Autodesk Inventor part; units mm, degrees
(part 2 of 4)
  line L562 (14.440387, 25.9675) -> (14.40122, 25.911667)
  line L563 (14.40122, 25.911667) -> (14.362054, 25.855)
  line L564 (14.362054, 25.855) -> (14.288721, 25.781667)
  line L565 (14.288721, 25.781667) -> (14.216221, 25.708334)
  line L566 (14.216221, 25.708334) -> (14.165388, 25.673334)
  line L567 (14.165388, 25.673334) -> (14.113721, 25.639168)
  line L568 (14.113721, 25.639168) -> (14.070388, 25.613335)
  line L569 (14.070388, 25.613335) -> (14.026222, 25.587501)
  line L570 (14.026222, 25.587501) -> (13.940389, 25.550835)
  line L571 (13.940389, 25.550835) -> (13.854556, 25.514168)
  line L572 (13.854556, 25.514168) -> (13.808722, 25.500835)
  line L573 (13.808722, 25.500835) -> (13.762056, 25.487501)
  line L574 (13.762056, 25.487501) -> (13.762056, 25.481668)
  line L575 (13.762056, 25.481668) -> (13.762056, 25.476668)
  line L576 (13.762056, 25.476668) -> (13.967889, 25.007504)
  line L577 (13.967889, 25.007504) -> (14.174555, 24.539171)
  line L578 (14.174555, 24.539171) -> (14.195388, 24.544171)
  line L579 (14.195388, 24.544171) -> (14.216221, 24.548337)
  line L580 (14.216221, 24.548337) -> (14.353721, 24.594171)
  line L581 (14.353721, 24.594171) -> (14.490387, 24.639171)
  line L582 (14.490387, 24.639171) -> (14.612053, 24.70167)
  line L583 (14.612053, 24.70167) -> (14.732886, 24.763337)
  line L584 (14.732886, 24.763337) -> (14.810386, 24.817503)
  line L585 (14.810386, 24.817503) -> (14.887052, 24.87167)
  line L586 (14.887052, 24.87167) -> (15.010385, 24.995003)
  line L587 (15.010385, 24.995003) -> (15.132885, 25.117502)
  line L588 (15.132885, 25.117502) -> (15.187885, 25.195002)
  line L589 (15.187885, 25.195002) -> (15.242051, 25.272502)
  line L590 (15.242051, 25.272502) -> (15.290384, 25.359168)
  line L591 (15.290384, 25.359168) -> (15.338717, 25.445834)
  line L592 (15.338717, 25.445834) -> (15.379551, 25.5475)
  line L593 (15.379551, 25.5475) -> (15.421217, 25.649167)
  line L594 (15.421217, 25.649167) -> (15.44955, 25.749999)
  line L595 (15.44955, 25.749999) -> (15.478717, 25.850832)
  line L596 (15.478717, 25.850832) -> (15.495383, 25.928332)
  line L597 (15.495383, 25.928332) -> (15.51205, 26.004998)
  line L598 (15.51205, 26.004998) -> (15.526217, 26.111665)
  line L599 (15.526217, 26.111665) -> (15.540383, 26.217497)
  line L600 (15.540383, 26.217497) -> (15.541217, 26.484163)
  line L601 (15.541217, 26.484163) -> (15.541217, 26.750829)
  line L602 (15.541217, 26.750829) -> (15.530383, 26.838329)
  line L603 (15.530383, 26.838329) -> (15.520383, 26.925829)
  line L604 (15.520383, 26.925829) -> (15.498717, 27.045828)
  line L605 (15.498717, 27.045828) -> (15.47705, 27.166661)
  line L606 (15.47705, 27.166661) -> (15.448717, 27.264994)
  line L607 (15.448717, 27.264994) -> (15.420384, 27.363327)
  line L608 (15.420384, 27.363327) -> (15.375384, 27.475827)
  line L609 (15.375384, 27.475827) -> (15.330384, 27.58916)
  line L610 (15.330384, 27.58916) -> (15.278717, 27.67916)
  line L611 (15.278717, 27.67916) -> (15.227051, 27.769993)
  line L612 (15.227051, 27.769993) -> (15.173718, 27.841659)
  line L613 (15.173718, 27.841659) -> (15.120385, 27.913325)
  line L614 (15.120385, 27.913325) -> (15.061218, 27.975825)
  line L615 (15.061218, 27.975825) -> (15.001218, 28.038325)
  line L616 (15.001218, 28.038325) -> (14.925385, 28.099158)
  line L617 (14.925385, 28.099158) -> (14.849552, 28.159991)
  line L618 (14.849552, 28.159991) -> (14.795385, 28.194158)
  line L619 (14.795385, 28.194158) -> (14.741219, 28.228324)
  line L620 (14.741219, 28.228324) -> (14.663719, 28.266657)
  line L621 (14.663719, 28.266657) -> (14.587053, 28.304991)
  line L622 (14.587053, 28.304991) -> (14.510387, 28.333324)
  line L623 (14.510387, 28.333324) -> (14.432887, 28.361657)
  line L624 (14.432887, 28.361657) -> (14.343721, 28.383324)
  line L625 (14.343721, 28.383324) -> (14.253721, 28.40499)
  line L626 (14.253721, 28.40499) -> (14.172054, 28.418324)
  line L627 (14.172054, 28.418324) -> (14.091221, 28.43249)
  line L628 (14.091221, 28.43249) -> (13.768721, 28.435823)
  line L629 (13.768721, 28.435823) -> (13.447056, 28.43999)
  line L630 (13.447056, 28.43999) -> (13.347889, 28.430823)
  line L631 (13.347889, 28.430823) -> (13.249556, 28.421657)
  line L632 (13.249556, 28.421657) -> (13.17039, 28.408324)
  line L633 (13.17039, 28.408324) -> (13.091223, 28.39499)
  line L634 (13.091223, 28.39499) -> (12.99539, 28.365824)
  line L635 (12.99539, 28.365824) -> (12.899557, 28.33749)
  line L636 (12.899557, 28.33749) -> (12.832891, 28.307491)
  line L637 (12.832891, 28.307491) -> (12.766225, 28.277491)
  line L638 (12.766225, 28.277491) -> (12.702058, 28.237491)
  line L639 (12.702058, 28.237491) -> (12.637892, 28.197491)
  line L640 (12.637892, 28.197491) -> (12.568725, 28.144991)
  line L641 (12.568725, 28.144991) -> (12.499559, 28.093325)
  line L642 (12.499559, 28.093325) -> (12.422059, 28.013325)
  line L643 (12.422059, 28.013325) -> (12.343726, 27.934158)
  line L644 (12.343726, 27.934158) -> (12.290393, 27.859159)
  line L645 (12.290393, 27.859159) -> (12.23706, 27.784159)
  line L646 (12.23706, 27.784159) -> (12.167893, 27.646659)
  line L647 (12.167893, 27.646659) -> (12.098727, 27.50916)
  line L648 (12.098727, 27.50916) -> (12.038727, 27.35916)
  line L649 (12.038727, 27.35916) -> (11.979561, 27.209161)
  line L650 (11.979561, 27.209161) -> (11.927894, 27.050828)
  line L651 (11.927894, 27.050828) -> (11.876228, 26.892495)
  line L652 (11.876228, 26.892495) -> (11.835395, 26.761662)
  line L653 (11.835395, 26.761662) -> (11.795395, 26.629996)
  line L654 (11.795395, 26.629996) -> (11.747895, 26.486663)
  line L655 (11.747895, 26.486663) -> (11.701229, 26.342497)
  line L656 (11.701229, 26.342497) -> (11.657895, 26.236664)
  line L657 (11.657895, 26.236664) -> (11.614562, 26.131664)
  line L658 (11.614562, 26.131664) -> (11.579562, 26.069998)
  line L659 (11.579562, 26.069998) -> (11.543729, 26.007498)
  line L660 (11.543729, 26.007498) -> (11.501229, 25.954165)
  line L661 (11.501229, 25.954165) -> (11.457896, 25.899998)
  line L662 (11.457896, 25.899998) -> (11.397063, 25.844999)
  line L663 (11.397063, 25.844999) -> (11.337063, 25.789165)
  line L664 (11.337063, 25.789165) -> (11.270397, 25.755832)
  line L665 (11.270397, 25.755832) -> (11.204563, 25.723332)
  line L666 (11.204563, 25.723332) -> (11.139563, 25.707499)
  line L667 (11.139563, 25.707499) -> (11.074564, 25.692499)
  line L668 (11.074564, 25.692499) -> (10.853731, 25.693332)
  line L669 (10.853731, 25.693332) -> (10.632898, 25.694166)
  line L670 (10.632898, 25.694166) -> (10.566232, 25.712499)
  line L671 (10.566232, 25.712499) -> (10.500399, 25.729999)
  line L672 (10.500399, 25.729999) -> (10.441232, 25.759999)
  line L673 (10.441232, 25.759999) -> (10.382899, 25.789999)
  line L674 (10.382899, 25.789999) -> (10.345399, 25.819999)
  line L675 (10.345399, 25.819999) -> (10.3079, 25.849999)
  line L676 (10.3079, 25.849999) -> (10.283733, 25.875832)
  line L677 (10.283733, 25.875832) -> (10.259566, 25.900832)
  line L678 (10.259566, 25.900832) -> (10.228733, 25.943332)
  line L679 (10.228733, 25.943332) -> (10.197067, 25.984998)
  line L680 (10.197067, 25.984998) -> (10.171233, 26.036665)
  line L681 (10.171233, 26.036665) -> (10.144567, 26.089164)
  line L682 (10.144567, 26.089164) -> (10.121233, 26.161664)
  line L683 (10.121233, 26.161664) -> (10.097067, 26.234164)
  line L684 (10.097067, 26.234164) -> (10.082067, 26.317497)
  line L685 (10.082067, 26.317497) -> (10.067067, 26.40083)
  line L686 (10.067067, 26.40083) -> (10.067067, 26.554996)
  line L687 (10.067067, 26.554996) -> (10.067067, 26.709162)
  line L688 (10.067067, 26.709162) -> (10.084567, 26.776662)
  line L689 (10.084567, 26.776662) -> (10.102067, 26.844162)
  line L690 (10.102067, 26.844162) -> (10.1229, 26.894995)
  line L691 (10.1229, 26.894995) -> (10.143733, 26.945828)
  line L692 (10.143733, 26.945828) -> (10.191233, 27.019161)
  line L693 (10.191233, 27.019161) -> (10.238733, 27.092495)
  line L694 (10.238733, 27.092495) -> (10.307066, 27.159161)
  line L695 (10.307066, 27.159161) -> (10.375399, 27.225827)
  line L696 (10.375399, 27.225827) -> (10.439565, 27.269994)
  line L697 (10.439565, 27.269994) -> (10.504565, 27.314994)
  line L698 (10.504565, 27.314994) -> (10.593732, 27.35916)
  line L699 (10.593732, 27.35916) -> (10.682898, 27.403327)
  line L700 (10.682898, 27.403327) -> (10.757898, 27.429993)
  line L701 (10.757898, 27.429993) -> (10.832065, 27.455827)
  line L702 (10.832065, 27.455827) -> (10.835398, 27.45916)
  line L703 (10.835398, 27.45916) -> (10.838731, 27.46166)
  line L704 (10.838731, 27.46166) -> (10.632899, 27.906657)
  line L705 (10.632899, 27.906657) -> (10.427066, 28.350823)
  line L706 (10.427066, 28.350823) -> (10.421233, 28.356657)
  line L707 (10.421233, 28.356657) -> (10.415399, 28.363323)
  line L708 (10.415399, 28.363323) -> (10.342066, 28.34249)
  line L709 (10.342066, 28.34249) -> (10.268733, 28.320823)
  line L710 (10.268733, 28.320823) -> (10.173733, 28.284157)
  line L711 (10.173733, 28.284157) -> (10.078733, 28.246657)
  line L712 (10.078733, 28.246657) -> (9.993734, 28.204157)
  line L713 (9.993734, 28.204157) -> (9.907901, 28.161658)
  line L714 (9.907901, 28.161658) -> (9.837067, 28.114991)
  line L715 (9.837067, 28.114991) -> (9.766234, 28.069158)
  line L716 (9.766234, 28.069158) -> (9.716234, 28.030825)
  line L717 (9.716234, 28.030825) -> (9.666234, 27.992492)
  line L718 (9.666234, 27.992492) -> (9.592068, 27.921658)
  line L719 (9.592068, 27.921658) -> (9.517902, 27.850825)
  line L720 (9.517902, 27.850825) -> (9.474568, 27.795825)
  line L721 (9.474568, 27.795825) -> (9.430402, 27.740825)
  line L722 (9.430402, 27.740825) -> (9.378735, 27.662492)
  line L723 (9.378735, 27.662492) -> (9.327069, 27.584159)
  line L724 (9.327069, 27.584159) -> (9.302903, 27.535826)
  line L725 (9.302903, 27.535826) -> (9.277903, 27.487493)
  line L726 (9.277903, 27.487493) -> (9.241236, 27.397493)
  line L727 (9.241236, 27.397493) -> (9.204569, 27.307493)
  line L728 (9.204569, 27.307493) -> (9.179569, 27.220827)
  line L729 (9.179569, 27.220827) -> (9.154569, 27.134161)
  line L730 (9.154569, 27.134161) -> (9.138736, 27.046661)
  line L731 (9.138736, 27.046661) -> (9.122069, 26.959161)
  line L732 (9.122069, 26.959161) -> (9.112903, 26.871662)
  line L733 (9.112903, 26.871662) -> (9.10457, 26.784162)
  line L734 (9.10457, 26.784162) -> (9.101236, 26.675829)
  line L735 (9.101236, 26.675829) -> (9.101239, 26.675831)
  line L736 (5.926259, 152.354502) -> (5.923571, 152.297378)
  line L737 (5.923571, 152.297378) -> (5.929619, 152.199933)
  line L738 (5.929619, 152.199933) -> (5.934996, 152.102487)
  line L739 (5.934996, 152.102487) -> (5.945076, 152.029906)
  line L740 (5.945076, 152.029906) -> (5.955829, 151.957326)
  line L741 (5.955829, 151.957326) -> (5.97263, 151.880041)
  line L742 (5.97263, 151.880041) -> (5.990103, 151.802757)
  line L743 (5.990103, 151.802757) -> (6.020345, 151.714047)
  line L744 (6.020345, 151.714047) -> (6.050587, 151.625338)
  line L745 (6.050587, 151.625338) -> (6.090237, 151.544693)
  line L746 (6.090237, 151.544693) -> (6.129215, 151.464048)
  line L747 (6.129215, 151.464048) -> (6.182978, 151.383403)
  line L748 (6.182978, 151.383403) -> (6.236742, 151.302758)
  line L749 (6.236742, 151.302758) -> (6.296553, 151.235554)
  line L750 (6.296553, 151.235554) -> (6.357037, 151.168349)
  line L751 (6.357037, 151.168349) -> (6.412144, 151.121307)
  line L752 (6.412144, 151.121307) -> (6.467252, 151.074936)
  line L753 (6.467252, 151.074936) -> (6.518999, 151.037974)
  line L754 (6.518999, 151.037974) -> (6.570746, 151.001683)
  line L755 (6.570746, 151.001683) -> (6.640638, 150.962705)
  line L756 (6.640638, 150.962705) -> (6.711202, 150.923727)
  line L757 (6.711202, 150.923727) -> (6.781767, 150.893485)
  line L758 (6.781767, 150.893485) -> (6.853003, 150.863915)
  line L759 (6.853003, 150.863915) -> (6.906766, 150.847114)
  line L760 (6.906766, 150.847114) -> (6.960529, 150.830313)
  line L761 (6.960529, 150.830313) -> (7.018997, 150.8162)
  line L762 (7.018997, 150.8162) -> (7.078136, 150.802087)
  line L763 (7.078136, 150.802087) -> (7.137276, 150.792007)
  line L764 (7.137276, 150.792007) -> (7.195744, 150.781926)
  line L765 (7.195744, 150.781926) -> (7.266308, 150.773189)
  line L766 (7.266308, 150.773189) -> (7.336872, 150.765125)
  line L767 (7.336872, 150.765125) -> (8.523024, 150.765125)
  line L768 (8.523024, 150.765125) -> (9.709176, 150.765125)
  line L769 (9.709176, 150.765125) -> (9.786461, 150.773862)
  line L770 (9.786461, 150.773862) -> (9.863745, 150.78327)
  line L771 (9.863745, 150.78327) -> (9.93767, 150.796039)
  line L772 (9.93767, 150.796039) -> (10.011594, 150.80948)
  line L773 (10.011594, 150.80948) -> (10.10232, 150.835689)
  line L774 (10.10232, 150.835689) -> (10.193717, 150.861899)
  line L775 (10.193717, 150.861899) -> (10.26697, 150.892813)
  line L776 (10.26697, 150.892813) -> (10.340222, 150.923726)
  line L777 (10.340222, 150.923726) -> (10.389281, 150.949936)
  line L778 (10.389281, 150.949936) -> (10.43834, 150.976817)
  line L779 (10.43834, 150.976817) -> (10.49748, 151.014452)
  line L780 (10.49748, 151.014452) -> (10.555947, 151.052758)
  line L781 (10.555947, 151.052758) -> (10.587533, 151.078296)
  line L782 (10.587533, 151.078296) -> (10.619791, 151.104505)
  line L783 (10.619791, 151.104505) -> (10.661457, 151.141467)
  line L784 (10.661457, 151.141467) -> (10.703796, 151.179102)
  line L785 (10.703796, 151.179102) -> (10.754199, 151.234881)
  line L786 (10.754199, 151.234881) -> (10.804602, 151.29066)
  line L787 (10.804602, 151.29066) -> (10.852989, 151.361225)
  line L788 (10.852989, 151.361225) -> (10.901376, 151.431789)
  line L789 (10.901376, 151.431789) -> (10.93901, 151.503697)
  line L790 (10.93901, 151.503697) -> (10.975972, 151.574934)
  line L791 (10.975972, 151.574934) -> (10.999494, 151.629369)
  line L792 (10.999494, 151.629369) -> (11.022343, 151.684476)
  line L793 (11.022343, 151.684476) -> (11.049897, 151.773857)
  line L794 (11.049897, 151.773857) -> (11.076778, 151.863911)
  line L795 (11.076778, 151.863911) -> (11.090219, 151.934475)
  line L796 (11.090219, 151.934475) -> (11.10366, 152.005039)
  line L797 (11.10366, 152.005039) -> (11.111725, 152.066867)
  line L798 (11.111725, 152.066867) -> (11.120461, 152.129367)
  line L799 (11.120461, 152.129367) -> (11.120461, 152.327619)
  line L800 (11.120461, 152.327619) -> (11.120461, 152.525871)
  line L801 (11.120461, 152.525871) -> (11.105004, 152.620629)
  line L802 (11.105004, 152.620629) -> (11.090219, 152.715386)
  line L803 (11.090219, 152.715386) -> (11.073418, 152.783935)
  line L804 (11.073418, 152.783935) -> (11.056617, 152.851811)
  line L805 (11.056617, 152.851811) -> (11.027047, 152.935816)
  line L806 (11.027047, 152.935816) -> (10.997477, 153.020493)
  line L807 (10.997477, 153.020493) -> (10.957155, 153.102482)
  line L808 (10.957155, 153.102482) -> (10.91616, 153.184471)
  line L809 (10.91616, 153.184471) -> (10.875166, 153.247643)
  line L810 (10.875166, 153.247643) -> (10.833499, 153.311487)
  line L811 (10.833499, 153.311487) -> (10.794521, 153.359202)
  line L812 (10.794521, 153.359202) -> (10.755543, 153.406917)
  line L813 (10.755543, 153.406917) -> (10.706484, 153.455976)
  line L814 (10.706484, 153.455976) -> (10.657425, 153.505035)
  line L815 (10.657425, 153.505035) -> (10.608365, 153.544685)
  line L816 (10.608365, 153.544685) -> (10.559306, 153.584336)
  line L817 (10.559306, 153.584336) -> (10.492774, 153.628018)
  line L818 (10.492774, 153.628018) -> (10.426242, 153.671701)
  line L819 (10.426242, 153.671701) -> (10.334845, 153.715384)
  line L820 (10.334845, 153.715384) -> (10.243447, 153.759066)
  line L821 (10.243447, 153.759066) -> (10.185652, 153.779228)
  line L822 (10.185652, 153.779228) -> (10.127184, 153.799389)
  line L823 (10.127184, 153.799389) -> (10.049228, 153.81955)
  line L824 (10.049228, 153.81955) -> (9.971271, 153.839711)
  line L825 (9.971271, 153.839711) -> (9.908771, 153.849792)
  line L826 (9.908771, 153.849792) -> (9.846944, 153.859872)
  line L827 (9.846944, 153.859872) -> (9.785116, 153.867937)
  line L828 (9.785116, 153.867937) -> (9.722616, 153.876001)
  line L829 (9.722616, 153.876001) -> (8.610388, 153.87869)
  line L830 (8.610388, 153.87869) -> (7.49816, 153.880706)
  line L831 (7.49816, 153.880706) -> (7.373833, 153.873313)
  line L832 (7.373833, 153.873313) -> (7.249505, 153.865921)
  line L833 (7.249505, 153.865921) -> (7.183645, 153.856512)
  line L834 (7.183645, 153.856512) -> (7.117785, 153.846432)
  line L835 (7.117785, 153.846432) -> (7.052597, 153.832319)
  line L836 (7.052597, 153.832319) -> (6.987409, 153.818206)
  line L837 (6.987409, 153.818206) -> (6.913485, 153.794685)
  line L838 (6.913485, 153.794685) -> (6.83956, 153.771163)
  line L839 (6.83956, 153.771163) -> (6.775716, 153.744282)
  line L840 (6.775716, 153.744282) -> (6.711872, 153.718072)
  line L841 (6.711872, 153.718072) -> (6.661469, 153.690518)
  line L842 (6.661469, 153.690518) -> (6.611066, 153.662965)
  line L843 (6.611066, 153.662965) -> (6.553943, 153.626002)
  line L844 (6.553943, 153.626002) -> (6.496819, 153.58904)
  line L845 (6.496819, 153.58904) -> (6.446416, 153.548046)
  line L846 (6.446416, 153.548046) -> (6.396013, 153.507051)
  line L847 (6.396013, 153.507051) -> (6.34561, 153.456648)
  line L848 (6.34561, 153.456648) -> (6.295207, 153.406245)
  line L849 (6.295207, 153.406245) -> (6.254213, 153.355842)
  line L850 (6.254213, 153.355842) -> (6.21389, 153.305439)
  line L851 (6.21389, 153.305439) -> (6.186336, 153.265116)
  line L852 (6.186336, 153.265116) -> (6.159455, 153.224794)
  line L853 (6.159455, 153.224794) -> (6.131229, 153.175735)
  line L854 (6.131229, 153.175735) -> (6.103003, 153.126676)
  line L855 (6.103003, 153.126676) -> (6.069401, 153.052751)
  line L856 (6.069401, 153.052751) -> (6.036471, 152.978155)
  line L857 (6.036471, 152.978155) -> (6.010262, 152.895494)
  line L858 (6.010262, 152.895494) -> (5.984052, 152.813505)
  line L859 (5.984052, 152.813505) -> (5.969267, 152.746973)
  line L860 (5.969267, 152.746973) -> (5.955154, 152.680441)
  line L861 (5.955154, 152.680441) -> (5.945746, 152.613237)
  line L862 (5.945746, 152.613237) -> (5.936337, 152.546033)
  line L863 (5.936337, 152.546033) -> (5.932305, 152.478829)
  line L864 (5.932305, 152.478829) -> (5.928945, 152.411625)
  line L865 (5.928945, 152.411625) -> (5.926257, 152.354501)
  line L866 (5.926257, 152.354501) -> (5.926259, 152.354502)
  line L867 (6.729349, 152.314852) -> (6.728677, 152.41297)
  line L868 (6.728677, 152.41297) -> (6.738757, 152.472781)
  line L869 (6.738757, 152.472781) -> (6.74951, 152.532593)
  line L870 (6.74951, 152.532593) -> (6.766983, 152.586356)
  line L871 (6.766983, 152.586356) -> (6.784456, 152.640119)
  line L872 (6.784456, 152.640119) -> (6.809994, 152.690522)
  line L873 (6.809994, 152.690522) -> (6.836203, 152.740925)
  line L874 (6.836203, 152.740925) -> (6.871821, 152.787968)
  line L875 (6.871821, 152.787968) -> (6.90744, 152.835011)
  line L876 (6.90744, 152.835011) -> (6.955827, 152.876005)
  line L877 (6.955827, 152.876005) -> (7.004886, 152.916328)
  line L878 (7.004886, 152.916328) -> (7.041176, 152.938505)
  line L879 (7.041176, 152.938505) -> (7.077466, 152.960683)
  line L880 (7.077466, 152.960683) -> (7.131229, 152.983532)
  line L881 (7.131229, 152.983532) -> (7.184992, 153.007053)
  line L882 (7.184992, 153.007053) -> (7.248164, 153.023182)
  line L883 (7.248164, 153.023182) -> (7.312008, 153.039311)
  line L884 (7.312008, 153.039311) -> (7.394669, 153.046704)
  line L885 (7.394669, 153.046704) -> (7.478002, 153.054096)
  line L886 (7.478002, 153.054096) -> (8.580149, 153.05208)
  line L887 (8.580149, 153.05208) -> (9.682296, 153.049392)
  line L888 (9.682296, 153.049392) -> (9.739419, 153.037295)
  line L889 (9.739419, 153.037295) -> (9.796543, 153.025871)
  line L890 (9.796543, 153.025871) -> (9.857026, 153.005709)
  line L891 (9.857026, 153.005709) -> (9.91751, 152.985548)
  line L892 (9.91751, 152.985548) -> (9.972618, 152.955978)
  line L893 (9.972618, 152.955978) -> (10.028397, 152.926408)
  line L894 (10.028397, 152.926408) -> (10.067375, 152.896838)
  line L895 (10.067375, 152.896838) -> (10.106354, 152.866597)
  line L896 (10.106354, 152.866597) -> (10.143316, 152.826946)
  line L897 (10.143316, 152.826946) -> (10.180278, 152.786624)
  line L898 (10.180278, 152.786624) -> (10.205144, 152.74899)
  line L899 (10.205144, 152.74899) -> (10.230682, 152.710683)
  line L900 (10.230682, 152.710683) -> (10.253531, 152.662296)
  line L901 (10.253531, 152.662296) -> (10.27638, 152.613237)
  line L902 (10.27638, 152.613237) -> (10.293181, 152.555442)
  line L903 (10.293181, 152.555442) -> (10.309982, 152.497646)
  line L904 (10.309982, 152.497646) -> (10.318047, 152.427754)
  line L905 (10.318047, 152.427754) -> (10.326111, 152.357862)
  line L906 (10.326111, 152.357862) -> (10.321407, 152.272513)
  line L907 (10.321407, 152.272513) -> (10.317375, 152.186492)
  line L908 (10.317375, 152.186492) -> (10.307294, 152.138105)
  line L909 (10.307294, 152.138105) -> (10.296542, 152.089046)
  line L910 (10.296542, 152.089046) -> (10.283773, 152.052083)
  line L911 (10.283773, 152.052083) -> (10.271004, 152.015121)
  line L912 (10.271004, 152.015121) -> (10.250843, 151.972783)
  line L913 (10.250843, 151.972783) -> (10.230009, 151.931116)
  line L914 (10.230009, 151.931116) -> (10.199096, 151.884073)
  line L915 (10.199096, 151.884073) -> (10.168182, 151.83703)
  line L916 (10.168182, 151.83703) -> (10.117779, 151.789316)
  line L917 (10.117779, 151.789316) -> (10.068048, 151.742273)
  line L918 (10.068048, 151.742273) -> (10.019661, 151.711359)
  line L919 (10.019661, 151.711359) -> (9.971946, 151.679773)
  line L920 (9.971946, 151.679773) -> (9.918183, 151.657596)
  line L921 (9.918183, 151.657596) -> (9.863748, 151.634746)
  line L922 (9.863748, 151.634746) -> (9.826785, 151.624666)
  line L923 (9.826785, 151.624666) -> (9.790495, 151.613913)
  line L924 (9.790495, 151.613913) -> (9.73942, 151.60316)
  line L925 (9.73942, 151.60316) -> (9.689017, 151.592408)
  line L926 (9.689017, 151.592408) -> (8.573429, 151.590392)
  line L927 (8.573429, 151.590392) -> (7.45784, 151.587703)
  line L928 (7.45784, 151.587703) -> (7.385932, 151.595096)
  line L929 (7.385932, 151.595096) -> (7.314023, 151.602488)
  line L930 (7.314023, 151.602488) -> (7.244803, 151.619289)
  line L931 (7.244803, 151.619289) -> (7.175583, 151.636762)
  line L932 (7.175583, 151.636762) -> (7.114427, 151.66566)
  line L933 (7.114427, 151.66566) -> (7.053272, 151.694558)
  line L934 (7.053272, 151.694558) -> (7.013621, 151.720768)
  line L935 (7.013621, 151.720768) -> (6.973971, 151.747649)
  line L936 (6.973971, 151.747649) -> (6.938353, 151.779907)
  line L937 (6.938353, 151.779907) -> (6.902734, 151.812165)
  line L938 (6.902734, 151.812165) -> (6.871149, 151.85316)
  line L939 (6.871149, 151.85316) -> (6.839563, 151.894154)
  line L940 (6.839563, 151.894154) -> (6.807977, 151.95531)
  line L941 (6.807977, 151.95531) -> (6.777063, 152.017138)
  line L942 (6.777063, 152.017138) -> (6.76295, 152.062836)
  line L943 (6.76295, 152.062836) -> (6.749509, 152.109207)
  line L944 (6.749509, 152.109207) -> (6.739429, 152.16297)
  line L945 (6.739429, 152.16297) -> (6.73002, 152.216733)
  line L946 (6.73002, 152.216733) -> (6.729348, 152.314851)
  line L947 (6.729348, 152.314851) -> (6.729349, 152.314852)
  line L948 (5.926259, 162.82489) -> (5.924243, 162.761046)
  line L949 (5.924243, 162.761046) -> (5.928947, 162.66696)
  line L950 (5.928947, 162.66696) -> (5.934324, 162.572875)
  line L951 (5.934324, 162.572875) -> (5.945076, 162.497606)
  line L952 (5.945076, 162.497606) -> (5.955829, 162.421666)
  line L953 (5.955829, 162.421666) -> (5.969942, 162.356477)
  line L954 (5.969942, 162.356477) -> (5.984055, 162.290618)
  line L955 (5.984055, 162.290618) -> (6.012952, 162.20258)
  line L956 (6.012952, 162.20258) -> (6.04185, 162.114543)
  line L957 (6.04185, 162.114543) -> (6.077468, 162.038602)
  line L958 (6.077468, 162.038602) -> (6.112415, 161.961989)
  line L959 (6.112415, 161.961989) -> (6.146016, 161.905538)
  line L960 (6.146016, 161.905538) -> (6.179619, 161.848414)
  line L961 (6.179619, 161.848414) -> (6.228678, 161.783226)
  line L962 (6.228678, 161.783226) -> (6.277065, 161.71871)
  line L963 (6.277065, 161.71871) -> (6.343597, 161.65285)
  line L964 (6.343597, 161.65285) -> (6.409457, 161.586318)
  line L965 (6.409457, 161.586318) -> (6.46322, 161.54398)
  line L966 (6.46322, 161.54398) -> (6.517655, 161.502313)
  line L967 (6.517655, 161.502313) -> (6.574107, 161.466695)
  line L968 (6.574107, 161.466695) -> (6.63123, 161.431749)
  line L969 (6.63123, 161.431749) -> (6.701794, 161.396803)
  line L970 (6.701794, 161.396803) -> (6.772359, 161.361857)
  line L971 (6.772359, 161.361857) -> (6.836203, 161.337663)
  line L972 (6.836203, 161.337663) -> (6.900719, 161.31347)
  line L973 (6.900719, 161.31347) -> (6.973971, 161.293309)
  line L974 (6.973971, 161.293309) -> (7.047895, 161.273148)
  line L975 (7.047895, 161.273148) -> (7.1319, 161.259035)
  line L976 (7.1319, 161.259035) -> (7.215906, 161.244922)
  line L977 (7.215906, 161.244922) -> (7.27975, 161.237529)
  line L978 (7.27975, 161.237529) -> (7.343593, 161.230137)
  line L979 (7.343593, 161.230137) -> (8.42222, 161.227449)
  line L980 (8.42222, 161.227449) -> (9.500846, 161.224761)
  line L981 (9.500846, 161.224761) -> (9.645335, 161.232153)
  line L982 (9.645335, 161.232153) -> (9.789823, 161.238873)
  line L983 (9.789823, 161.238873) -> (9.859043, 161.248954)
  line L984 (9.859043, 161.248954) -> (9.928263, 161.259035)
  line L985 (9.928263, 161.259035) -> (10.005548, 161.275836)
  line L986 (10.005548, 161.275836) -> (10.082161, 161.292637)
  line L987 (10.082161, 161.292637) -> (10.16415, 161.319518)
  line L988 (10.16415, 161.319518) -> (10.246811, 161.347072)
  line L989 (10.246811, 161.347072) -> (10.342913, 161.393443)
  line L990 (10.342913, 161.393443) -> (10.438342, 161.440486)
  line L991 (10.438342, 161.440486) -> (10.50017, 161.48148)
  line L992 (10.50017, 161.48148) -> (10.561326, 161.521803)
  line L993 (10.561326, 161.521803) -> (10.611729, 161.563469)
  line L994 (10.611729, 161.563469) -> (10.662132, 161.605135)
  line L995 (10.662132, 161.605135) -> (10.725304, 161.670324)
  line L996 (10.725304, 161.670324) -> (10.787803, 161.736183)
  line L997 (10.787803, 161.736183) -> (10.830814, 161.793979)
  line L998 (10.830814, 161.793979) -> (10.873153, 161.851774)
  line L999 (10.873153, 161.851774) -> (10.914819, 161.923683)
  line L1000 (10.914819, 161.923683) -> (10.955814, 161.995591)
  line L1001 (10.955814, 161.995591) -> (10.986055, 162.064139)
  line L1002 (10.986055, 162.064139) -> (11.016297, 162.132688)
  line L1003 (11.016297, 162.132688) -> (11.03713, 162.198548)
  line L1004 (11.03713, 162.198548) -> (11.057964, 162.263736)
  line L1005 (11.057964, 162.263736) -> (11.074093, 162.326235)
  line L1006 (11.074093, 162.326235) -> (11.090221, 162.388735)
  line L1007 (11.090221, 162.388735) -> (11.105006, 162.484165)
  line L1008 (11.105006, 162.484165) -> (11.120463, 162.579595)
  line L1009 (11.120463, 162.579595) -> (11.120463, 162.771127)
  line L1010 (11.120463, 162.771127) -> (11.120463, 162.962658)
  line L1011 (11.120463, 162.962658) -> (11.109039, 163.053384)
  line L1012 (11.109039, 163.053384) -> (11.096942, 163.144109)
  line L1013 (11.096942, 163.144109) -> (11.078797, 163.221394)
  line L1014 (11.078797, 163.221394) -> (11.05998, 163.298678)
  line L1015 (11.05998, 163.298678) -> (11.035114, 163.376635)
  line L1016 (11.035114, 163.376635) -> (11.010921, 163.455264)
  line L1017 (11.010921, 163.455264) -> (10.97463, 163.531205)
  line L1018 (10.97463, 163.531205) -> (10.93834, 163.607817)
  line L1019 (10.93834, 163.607817) -> (10.910114, 163.656876)
  line L1020 (10.910114, 163.656876) -> (10.881889, 163.705263)
  line L1021 (10.881889, 163.705263) -> (10.846271, 163.754994)
  line L1022 (10.846271, 163.754994) -> (10.811324, 163.804725)
  line L1023 (10.811324, 163.804725) -> (10.769658, 163.854456)
  line L1024 (10.769658, 163.854456) -> (10.728663, 163.903515)
  line L1025 (10.728663, 163.903515) -> (10.658771, 163.966687)
  line L1026 (10.658771, 163.966687) -> (10.589551, 164.029187)
  line L1027 (10.589551, 164.029187) -> (10.510922, 164.082278)
  line L1028 (10.510922, 164.082278) -> (10.431622, 164.135369)
  line L1029 (10.431622, 164.135369) -> (10.349633, 164.17502)
  line L1030 (10.349633, 164.17502) -> (10.266972, 164.215342)
  line L1031 (10.266972, 164.215342) -> (10.201112, 164.239536)
  line L1032 (10.201112, 164.239536) -> (10.135924, 164.263057)
  line L1033 (10.135924, 164.263057) -> (10.058639, 164.283218)
  line L1034 (10.058639, 164.283218) -> (9.981355, 164.30338)
  line L1035 (9.981355, 164.30338) -> (9.90071, 164.31682)
  line L1036 (9.90071, 164.31682) -> (9.820065, 164.330261)
  line L1037 (9.820065, 164.330261) -> (9.724635, 164.337654)
  line L1038 (9.724635, 164.337654) -> (9.628533, 164.344374)
  line L1039 (9.628533, 164.344374) -> (8.459183, 164.341686)
  line L1040 (8.459183, 164.341686) -> (7.289833, 164.338998)
  line L1041 (7.289833, 164.338998) -> (7.217252, 164.327573)
  line L1042 (7.217252, 164.327573) -> (7.144672, 164.31682)
  line L1043 (7.144672, 164.31682) -> (7.064027, 164.300019)
  line L1044 (7.064027, 164.300019) -> (6.984054, 164.283218)
  line L1045 (6.984054, 164.283218) -> (6.888624, 164.251633)
  line L1046 (6.888624, 164.251633) -> (6.793866, 164.220719)
  line L1047 (6.793866, 164.220719) -> (6.701125, 164.174348)
  line L1048 (6.701125, 164.174348) -> (6.607711, 164.128649)
  line L1049 (6.607711, 164.128649) -> (6.542523, 164.084295)
  line L1050 (6.542523, 164.084295) -> (6.476663, 164.03994)
  line L1051 (6.476663, 164.03994) -> (6.4229, 163.994241)
  line L1052 (6.4229, 163.994241) -> (6.369137, 163.948542)
  line L1053 (6.369137, 163.948542) -> (6.328814, 163.905532)
  line L1054 (6.328814, 163.905532) -> (6.28782, 163.863193)
  line L1055 (6.28782, 163.863193) -> (6.250186, 163.816151)
  line L1056 (6.250186, 163.816151) -> (6.213223, 163.769108)
  line L1057 (6.213223, 163.769108) -> (6.179621, 163.718705)
  line L1058 (6.179621, 163.718705) -> (6.145347, 163.668302)
  line L1059 (6.145347, 163.668302) -> (6.115106, 163.611178)
  line L1060 (6.115106, 163.611178) -> (6.084192, 163.554055)
  line L1061 (6.084192, 163.554055) -> (6.053278, 163.48013)
  line L1062 (6.053278, 163.48013) -> (6.022364, 163.406878)
  line L1063 (6.022364, 163.406878) -> (6.000187, 163.329593)
  line L1064 (6.000187, 163.329593) -> (5.977337, 163.251637)
  line L1065 (5.977337, 163.251637) -> (5.963896, 163.181072)
  line L1066 (5.963896, 163.181072) -> (5.949784, 163.110508)
  line L1067 (5.949784, 163.110508) -> (5.943063, 163.063465)
  line L1068 (5.943063, 163.063465) -> (5.936343, 163.016422)
  line L1069 (5.936343, 163.016422) -> (5.932983, 162.952579)
  line L1070 (5.932983, 162.952579) -> (5.92895, 162.888735)
  line L1071 (5.92895, 162.888735) -> (5.926262, 162.824891)
  line L1072 (5.926262, 162.824891) -> (5.926259, 162.82489)
  line L1073 (6.729349, 162.778519) -> (6.728677, 162.876637)
  line L1074 (6.728677, 162.876637) -> (6.738757, 162.936449)
  line L1075 (6.738757, 162.936449) -> (6.74951, 162.996261)
  line L1076 (6.74951, 162.996261) -> (6.763623, 163.043303)
  line L1077 (6.763623, 163.043303) -> (6.777064, 163.090346)
  line L1078 (6.777064, 163.090346) -> (6.805961, 163.14747)
  line L1079 (6.805961, 163.14747) -> (6.834859, 163.204593)
  line L1080 (6.834859, 163.204593) -> (6.866445, 163.24626)
  line L1081 (6.866445, 163.24626) -> (6.898031, 163.288598)
  line L1082 (6.898031, 163.288598) -> (6.944402, 163.330937)
  line L1083 (6.944402, 163.330937) -> (6.990773, 163.373275)
  line L1084 (6.990773, 163.373275) -> (7.043192, 163.404189)
  line L1085 (7.043192, 163.404189) -> (7.094939, 163.435103)
  line L1086 (7.094939, 163.435103) -> (7.155423, 163.458624)
  line L1087 (7.155423, 163.458624) -> (7.215907, 163.482818)
  line L1088 (7.215907, 163.482818) -> (7.283111, 163.498275)
  line L1089 (7.283111, 163.498275) -> (7.350315, 163.51306)
  line L1090 (7.350315, 163.51306) -> (8.479342, 163.515748)
  line L1091 (8.479342, 163.515748) -> (9.60837, 163.517764)
  line L1092 (9.60837, 163.517764) -> (9.674902, 163.510372)
  line L1093 (9.674902, 163.510372) -> (9.742106, 163.502307)
  line L1094 (9.742106, 163.502307) -> (9.803262, 163.48685)
  line L1095 (9.803262, 163.48685) -> (9.864417, 163.471393)
  line L1096 (9.864417, 163.471393) -> (9.916837, 163.449888)
  line L1097 (9.916837, 163.449888) -> (9.968584, 163.428383)
  line L1098 (9.968584, 163.428383) -> (10.020331, 163.394781)
  line L1099 (10.020331, 163.394781) -> (10.072078, 163.360507)
  line L1100 (10.072078, 163.360507) -> (10.117777, 163.316152)
  line L1101 (10.117777, 163.316152) -> (10.164148, 163.271797)
  line L1102 (10.164148, 163.271797) -> (10.193717, 163.230803)
  line L1103 (10.193717, 163.230803) -> (10.223287, 163.189136)
  line L1104 (10.223287, 163.189136) -> (10.253529, 163.12462)
  line L1105 (10.253529, 163.12462) -> (10.283771, 163.060104)
  line L1106 (10.283771, 163.060104) -> (10.297212, 163.006341)
  line L1107 (10.297212, 163.006341) -> (10.310652, 162.952578)
  line L1108 (10.310652, 162.952578) -> (10.317373, 162.89747)
  line L1109 (10.317373, 162.89747) -> (10.324093, 162.842363)
  line L1110 (10.324093, 162.842363) -> (10.324093, 162.784568)
  line L1111 (10.324093, 162.784568) -> (10.324093, 162.726772)
  line L1112 (10.324093, 162.726772) -> (10.317373, 162.672337)
  line L1113 (10.317373, 162.672337) -> (10.310652, 162.617902)
  line L1114 (10.310652, 162.617902) -> (10.297212, 162.566827)
  line L1115 (10.297212, 162.566827) -> (10.284443, 162.516424)
  line L1116 (10.284443, 162.516424) -> (10.26361, 162.465349)
  line L1117 (10.26361, 162.465349) -> (10.242104, 162.414274)
  line L1118 (10.242104, 162.414274) -> (10.210518, 162.365887)
  line L1119 (10.210518, 162.365887) -> (10.17826, 162.3175)
  line L1120 (10.17826, 162.3175) -> (10.14533, 162.281209)
  line L1121 (10.14533, 162.281209) -> (10.1124, 162.244247)
  line L1122 (10.1124, 162.244247) -> (10.058637, 162.204597)
  line L1123 (10.058637, 162.204597) -> (10.004874, 162.164274)
  line L1124 (10.004874, 162.164274) -> (9.942374, 162.134704)
  line L1125 (9.942374, 162.134704) -> (9.880546, 162.105134)
  line L1126 (9.880546, 162.105134) -> (9.803934, 162.085645)
  line L1127 (9.803934, 162.085645) -> (9.727321, 162.066156)
  line L1128 (9.727321, 162.066156) -> (9.647348, 162.059435)
  line L1129 (9.647348, 162.059435) -> (9.568047, 162.052043)
  line L1130 (9.568047, 162.052043) -> (8.523023, 162.052043)
  line L1131 (8.523023, 162.052043) -> (7.477998, 162.052043)
  line L1132 (7.477998, 162.052043) -> (7.400713, 162.058763)
  line L1133 (7.400713, 162.058763) -> (7.323429, 162.065484)
  line L1134 (7.323429, 162.065484) -> (7.255553, 162.082285)
  line L1135 (7.255553, 162.082285) -> (7.187677, 162.099086)
  line L1136 (7.187677, 162.099086) -> (7.14601, 162.115887)
  line L1137 (7.14601, 162.115887) -> (7.104344, 162.132016)
  line L1138 (7.104344, 162.132016) -> (7.060661, 162.156209)
  line L1139 (7.060661, 162.156209) -> (7.01765, 162.180403)
  line L1140 (7.01765, 162.180403) -> (6.96792, 162.220053)
  line L1141 (6.96792, 162.220053) -> (6.91886, 162.259704)
  line L1142 (6.91886, 162.259704) -> (6.885258, 162.30137)
  line L1143 (6.885258, 162.30137) -> (6.851656, 162.342365)
  line L1144 (6.851656, 162.342365) -> (6.822759, 162.392768)
  line L1145 (6.822759, 162.392768) -> (6.793861, 162.443171)
  line L1146 (6.793861, 162.443171) -> (6.771683, 162.507687)
  line L1147 (6.771683, 162.507687) -> (6.749506, 162.572875)
  line L1148 (6.749506, 162.572875) -> (6.739425, 162.626638)
  line L1149 (6.739425, 162.626638) -> (6.730017, 162.680401)
  line L1150 (6.730017, 162.680401) -> (6.729345, 162.778519)
  line L1151 (6.729345, 162.778519) -> (6.729349, 162.778519)
  line L1152 (8.831224, -33.4262) -> (8.829557, -33.806199)
  line L1153 (8.829557, -33.806199) -> (8.868724, -33.819532)
  line L1154 (8.868724, -33.819532) -> (8.908724, -33.832866)
  line L1155 (8.908724, -33.832866) -> (12.008714, -34.778697)
  line L1156 (12.008714, -34.778697) -> (15.108705, -35.725359)
  line L1157 (15.108705, -35.725359) -> (15.132038, -35.730359)
  line L1158 (15.132038, -35.730359) -> (15.154538, -35.735359)
  line L1159 (15.154538, -35.735359) -> (15.152872, -35.207027)
  line L1160 (15.152872, -35.207027) -> (15.150372, -34.678694)
  line L1161 (15.150372, -34.678694) -> (14.575374, -34.522861)
  line L1162 (14.575374, -34.522861) -> (14.000377, -34.367028)
  line L1163 (14.000377, -34.367028) -> (13.98121, -34.362028)
  line L1164 (13.98121, -34.362028) -> (13.962877, -34.357862)
  line L1165 (13.962877, -34.357862) -> (13.962877, -33.426197)
  line L1166 (13.962877, -33.426197) -> (13.962877, -32.494533)
  line L1167 (13.962877, -32.494533) -> (14.544542, -32.337034)
  line L1168 (14.544542, -32.337034) -> (15.125372, -32.180367)
  line L1169 (15.125372, -32.180367) -> (15.139539, -32.172867)
  line L1170 (15.139539, -32.172867) -> (15.154539, -32.165367)
  line L1171 (15.154539, -32.165367) -> (15.154539, -31.645369)
  line L1172 (15.154539, -31.645369) -> (15.154539, -31.12537)
  line L1173 (15.154539, -31.12537) -> (15.148706, -31.122036)
  line L1174 (15.148706, -31.122036) -> (15.142039, -31.118703)
  line L1175 (15.142039, -31.118703) -> (11.987872, -32.082868)
  line L1176 (11.987872, -32.082868) -> (8.833705, -33.046198)
  line L1177 (8.833705, -33.046198) -> (8.831205, -33.426198)
  line L1178 (8.831205, -33.426198) -> (8.831224, -33.4262)
  line L1179 (10.539551, -33.425366) -> (10.550385, -33.4212)
  line L1180 (10.550385, -33.4212) -> (11.779547, -33.087034)
  line L1181 (11.779547, -33.087034) -> (13.00871, -32.752867)
  line L1182 (13.00871, -32.752867) -> (13.01121, -33.423697)
  line L1183 (13.01121, -33.423697) -> (13.012877, -34.093696)
  line L1184 (13.012877, -34.093696) -> (13.010377, -34.096196)
  line L1185 (13.010377, -34.096196) -> (13.007877, -34.099529)
  line L1186 (13.007877, -34.099529) -> (11.76788, -33.764532)
  line L1187 (11.76788, -33.764532) -> (10.527882, -33.429534)
  line L1188 (10.527882, -33.429534) -> (10.539549, -33.425367)
  line L1189 (10.539549, -33.425367) -> (10.539551, -33.425366)
  line L1190 (8.831224, -29.289547) -> (8.829557, -30.44121)
  line L1191 (8.829557, -30.44121) -> (11.987882, -30.44121)
  line L1192 (11.987882, -30.44121) -> (15.146206, -30.44121)
  line L1193 (15.146206, -30.44121) -> (15.146206, -29.941211)
  line L1194 (15.146206, -29.941211) -> (15.146206, -29.441212)
  line L1195 (15.146206, -29.441212) -> (13.829544, -29.441212)
  line L1196 (13.829544, -29.441212) -> (12.512882, -29.441212)
  line L1197 (12.512882, -29.441212) -> (12.512882, -29.05538)
  line L1198 (12.512882, -29.05538) -> (12.512882, -28.670383)
  line L1199 (12.512882, -28.670383) -> (13.829544, -28.124551)
  line L1200 (13.829544, -28.124551) -> (15.145375, -27.578719)
  line L1201 (15.145375, -27.578719) -> (15.146208, -27.004553)
  line L1202 (15.146208, -27.004553) -> (15.146208, -26.431222)
  line L1203 (15.146208, -26.431222) -> (15.133708, -26.436222)
  line L1204 (15.133708, -26.436222) -> (15.121208, -26.441222)
  line L1205 (15.121208, -26.441222) -> (13.757047, -27.040386)
  line L1206 (13.757047, -27.040386) -> (12.393717, -27.640385)
  line L1207 (12.393717, -27.640385) -> (12.355384, -27.551218)
  line L1208 (12.355384, -27.551218) -> (12.317051, -27.462052)
  line L1209 (12.317051, -27.462052) -> (12.267051, -27.379552)
  line L1210 (12.267051, -27.379552) -> (12.217051, -27.297052)
  line L1211 (12.217051, -27.297052) -> (12.175385, -27.242052)
  line L1212 (12.175385, -27.242052) -> (12.133719, -27.187053)
  line L1213 (12.133719, -27.187053) -> (12.037052, -27.09122)
  line L1214 (12.037052, -27.09122) -> (11.939553, -26.995387)
  line L1215 (11.939553, -26.995387) -> (11.870386, -26.947054)
  line L1216 (11.870386, -26.947054) -> (11.800386, -26.899554)
  line L1217 (11.800386, -26.899554) -> (11.737887, -26.863721)
  line L1218 (11.737887, -26.863721) -> (11.675387, -26.828721)
  line L1219 (11.675387, -26.828721) -> (11.602054, -26.797887)
  line L1220 (11.602054, -26.797887) -> (11.528721, -26.766221)
  line L1221 (11.528721, -26.766221) -> (11.443721, -26.740388)
  line L1222 (11.443721, -26.740388) -> (11.358721, -26.713721)
  line L1223 (11.358721, -26.713721) -> (11.282055, -26.697054)
  line L1224 (11.282055, -26.697054) -> (11.204555, -26.680388)
  line L1225 (11.204555, -26.680388) -> (11.086222, -26.667054)
  line L1226 (11.086222, -26.667054) -> (10.967056, -26.653721)
  line L1227 (10.967056, -26.653721) -> (10.629557, -26.655388)
  line L1228 (10.629557, -26.655388) -> (10.292059, -26.657054)
  line L1229 (10.292059, -26.657054) -> (10.219559, -26.666221)
  line L1230 (10.219559, -26.666221) -> (10.147059, -26.675388)
  line L1231 (10.147059, -26.675388) -> (10.068726, -26.692054)
  line L1232 (10.068726, -26.692054) -> (9.990393, -26.707888)
  line L1233 (9.990393, -26.707888) -> (9.916227, -26.728721)
  line L1234 (9.916227, -26.728721) -> (9.84206, -26.750387)
  line L1235 (9.84206, -26.750387) -> (9.750394, -26.787887)
  line L1236 (9.750394, -26.787887) -> (9.658728, -26.825387)
  line L1237 (9.658728, -26.825387) -> (9.576228, -26.872887)
  line L1238 (9.576228, -26.872887) -> (9.493728, -26.92122)
  line L1239 (9.493728, -26.92122) -> (9.422062, -26.975386)
  line L1240 (9.422062, -26.975386) -> (9.350396, -27.030386)
  line L1241 (9.350396, -27.030386) -> (9.275396, -27.106219)
  line L1242 (9.275396, -27.106219) -> (9.200396, -27.182053)
  line L1243 (9.200396, -27.182053) -> (9.152896, -27.246219)
  line L1244 (9.152896, -27.246219) -> (9.10623, -27.310386)
  line L1245 (9.10623, -27.310386) -> (9.075397, -27.361219)
  line L1246 (9.075397, -27.361219) -> (9.045397, -27.412052)
  line L1247 (9.045397, -27.412052) -> (9.00873, -27.487052)
  line L1248 (9.00873, -27.487052) -> (8.972897, -27.562052)
  line L1249 (8.972897, -27.562052) -> (8.942897, -27.643718)
  line L1250 (8.942897, -27.643718) -> (8.912064, -27.726218)
  line L1251 (8.912064, -27.726218) -> (8.887064, -27.831218)
  line L1252 (8.887064, -27.831218) -> (8.862064, -27.937051)
  line L1253 (8.862064, -27.937051) -> (8.847897, -28.03705)
  line L1254 (8.847897, -28.03705) -> (8.833731, -28.13705)
  line L1255 (8.833731, -28.13705) -> (8.831231, -29.289546)
  line L1256 (8.831231, -29.289546) -> (8.831224, -29.289547)
  line L1257 (9.790387, -28.817881) -> (9.792887, -28.195382)
  line L1258 (9.792887, -28.195382) -> (9.807887, -28.145382)
  line L1259 (9.807887, -28.145382) -> (9.822887, -28.095382)
  line L1260 (9.822887, -28.095382) -> (9.851221, -28.037049)
  line L1261 (9.851221, -28.037049) -> (9.880387, -27.978716)
  line L1262 (9.880387, -27.978716) -> (9.915387, -27.933716)
  line L1263 (9.915387, -27.933716) -> (9.950387, -27.887883)
  line L1264 (9.950387, -27.887883) -> (10.000387, -27.847049)
  line L1265 (10.000387, -27.847049) -> (10.050387, -27.807049)
  line L1266 (10.050387, -27.807049) -> (10.125387, -27.770383)
  line L1267 (10.125387, -27.770383) -> (10.200386, -27.733716)
  line L1268 (10.200386, -27.733716) -> (10.262886, -27.717049)
  line L1269 (10.262886, -27.717049) -> (10.325386, -27.69955)
  line L1270 (10.325386, -27.69955) -> (10.417052, -27.691216)
  line L1271 (10.417052, -27.691216) -> (10.508718, -27.683716)
  line L1272 (10.508718, -27.683716) -> (10.679551, -27.683716)
  line L1273 (10.679551, -27.683716) -> (10.850384, -27.683716)
  line L1274 (10.850384, -27.683716) -> (10.935384, -27.691216)
  line L1275 (10.935384, -27.691216) -> (11.01955, -27.698716)
  line L1276 (11.01955, -27.698716) -> (11.072883, -27.712049)
  line L1277 (11.072883, -27.712049) -> (11.125383, -27.725383)
  line L1278 (11.125383, -27.725383) -> (11.17955, -27.746216)
  line L1279 (11.17955, -27.746216) -> (11.233716, -27.767883)
  line L1280 (11.233716, -27.767883) -> (11.288716, -27.804549)
  line L1281 (11.288716, -27.804549) -> (11.344549, -27.841216)
  line L1282 (11.344549, -27.841216) -> (11.394549, -27.895383)
  line L1283 (11.394549, -27.895383) -> (11.445382, -27.948716)
  line L1284 (11.445382, -27.948716) -> (11.478716, -28.017882)
  line L1285 (11.478716, -28.017882) -> (11.512882, -28.087049)
  line L1286 (11.512882, -28.087049) -> (11.531215, -28.153715)
  line L1287 (11.531215, -28.153715) -> (11.549549, -28.220381)
  line L1288 (11.549549, -28.220381) -> (11.552882, -28.831212)
  line L1289 (11.552882, -28.831212) -> (11.555382, -29.44121)
  line L1290 (11.555382, -29.44121) -> (10.671217, -29.44121)
  line L1291 (10.671217, -29.44121) -> (9.787052, -29.44121)
  line L1292 (9.787052, -29.44121) -> (9.790385, -28.817879)
  line L1293 (9.790385, -28.817879) -> (9.790387, -28.817881)
  line L1294 (8.829555, -25.010406) -> (8.829555, -25.532905)
  line L1295 (8.829555, -25.532905) -> (11.992037, -25.532905)
  line L1296 (11.992037, -25.532905) -> (15.154518, -25.532905)
  line L1297 (15.154518, -25.532905) -> (15.154518, -25.066242)
  line L1298 (15.154518, -25.066242) -> (15.154518, -24.599578)
  line L1299 (15.154518, -24.599578) -> (13.092025, -24.597911)
  line L1300 (13.092025, -24.597911) -> (11.030366, -24.595411)
  line L1301 (11.030366, -24.595411) -> (12.622861, -24.038748)
  line L1302 (12.622861, -24.038748) -> (14.21619, -23.482916)
  line L1303 (14.21619, -23.482916) -> (14.21869, -23.480416)
  line L1304 (14.21869, -23.480416) -> (14.22119, -23.477083)
  line L1305 (14.22119, -23.477083) -> (14.22119, -23.135417)
  line L1306 (14.22119, -23.135417) -> (14.22119, -22.792917)
  line L1307 (14.22119, -22.792917) -> (14.022857, -22.725417)
  line L1308 (14.022857, -22.725417) -> (13.825357, -22.657084)
  line L1309 (13.825357, -22.657084) -> (12.371196, -22.162087)
  line L1310 (12.371196, -22.162087) -> (10.917036, -21.667089)
  line L1311 (10.917036, -21.667089) -> (13.033696, -21.664589)
  line L1312 (13.033696, -21.664589) -> (15.150356, -21.662089)
  line L1313 (15.150356, -21.662089) -> (15.152856, -21.201259)
  line L1314 (15.152856, -21.201259) -> (15.154523, -20.74126)
  line L1315 (15.154523, -20.74126) -> (11.992041, -20.74126)
  line L1316 (11.992041, -20.74126) -> (8.829559, -20.74126)
  line L1317 (8.829559, -20.74126) -> (8.829559, -21.261259)
  line L1318 (8.829559, -21.261259) -> (8.829559, -21.781258)
  line L1319 (8.829559, -21.781258) -> (9.052892, -21.857091)
  line L1320 (9.052892, -21.857091) -> (9.275391, -21.933757)
  line L1321 (9.275391, -21.933757) -> (11.026219, -22.535422)
  line L1322 (11.026219, -22.535422) -> (12.776212, -23.137087)
  line L1323 (12.776212, -23.137087) -> (10.809552, -23.806251)
  line L1324 (10.809552, -23.806251) -> (8.84206, -24.475415)
  line L1325 (8.84206, -24.475415) -> (8.836226, -24.482082)
  line L1326 (8.836226, -24.482082) -> (8.82956, -24.487915)
  line L1327 (8.82956, -24.487915) -> (8.82956, -25.010415)
  line L1328 (8.82956, -25.010415) -> (8.829555, -25.010406)
  line L1329 (9.162058, -2.619858) -> (9.162058, -4.536519)
  line L1330 (9.162058, -4.536519) -> (9.641222, -4.536519)
  line L1331 (9.641222, -4.536519) -> (10.120386, -4.536519)
  line L1332 (10.120386, -4.536519) -> (10.120386, -3.828186)
  line L1333 (10.120386, -3.828186) -> (10.120386, -3.119854)
  line L1334 (10.120386, -3.119854) -> (12.802044, -3.118187)
  line L1335 (12.802044, -3.118187) -> (15.48287, -3.115687)
  line L1336 (15.48287, -3.115687) -> (15.48287, -2.615688)
  line L1337 (15.48287, -2.615688) -> (15.48287, -2.115689)
  line L1338 (15.48287, -2.115689) -> (12.802044, -2.113189)
  line L1339 (12.802044, -2.113189) -> (10.120386, -2.111523)
  line L1340 (10.120386, -2.111523) -> (10.120386, -1.407357)
  line L1341 (10.120386, -1.407357) -> (10.120386, -0.703192)
  line L1342 (10.120386, -0.703192) -> (9.641222, -0.703192)
  line L1343 (9.641222, -0.703192) -> (9.162058, -0.703192)
  line L1344 (9.162058, -0.703192) -> (9.162058, -2.619852)
  line L1345 (9.162058, -2.619852) -> (9.162058, -2.619858)
  line L1346 (9.161239, 5.598393) -> (9.162072, 4.571731)
  line L1347 (9.162072, 4.571731) -> (12.324554, 4.571731)
  line L1348 (12.324554, 4.571731) -> (15.487036, 4.571731)
  line L1349 (15.487036, 4.571731) -> (15.487036, 5.07173)
  line L1350 (15.487036, 5.07173) -> (15.487036, 5.571729)
  line L1351 (15.487036, 5.571729) -> (14.262874, 5.571729)
  line L1352 (14.262874, 5.571729) -> (13.038713, 5.571729)
  line L1353 (13.038713, 5.571729) -> (13.034546, 6.206726)
  line L1354 (13.034546, 6.206726) -> (13.029546, 6.842558)
  line L1355 (13.029546, 6.842558) -> (13.02038, 6.915891)
  line L1356 (13.02038, 6.915891) -> (13.01038, 6.98839)
  line L1357 (13.01038, 6.98839) -> (12.99038, 7.08839)
  line L1358 (12.99038, 7.08839) -> (12.97038, 7.18839)
  line L1359 (12.97038, 7.18839) -> (12.933713, 7.29839)
  line L1360 (12.933713, 7.29839) -> (12.897047, 7.409223)
  line L1361 (12.897047, 7.409223) -> (12.839547, 7.520055)
  line L1362 (12.839547, 7.520055) -> (12.78288, 7.630888)
  line L1363 (12.78288, 7.630888) -> (12.741214, 7.690055)
  line L1364 (12.741214, 7.690055) -> (12.699548, 7.749221)
  line L1365 (12.699548, 7.749221) -> (12.661215, 7.795888)
  line L1366 (12.661215, 7.795888) -> (12.623715, 7.842554)
  line L1367 (12.623715, 7.842554) -> (12.538715, 7.92172)
  line L1368 (12.538715, 7.92172) -> (12.454548, 8.000887)
  line L1369 (12.454548, 8.000887) -> (12.398715, 8.03922)
  line L1370 (12.398715, 8.03922) -> (12.343715, 8.078387)
  line L1371 (12.343715, 8.078387) -> (12.277882, 8.115886)